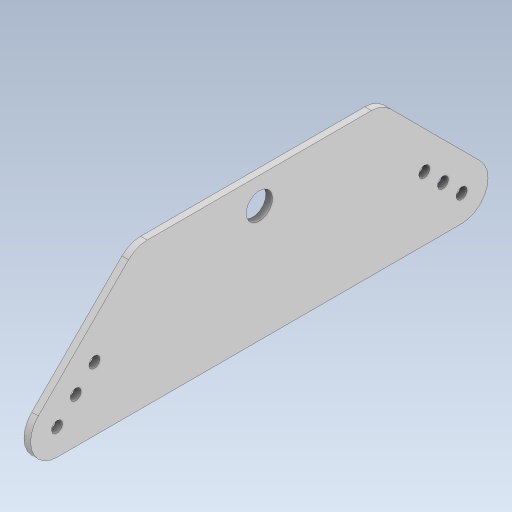
# Autodesk Inventor part: HipPivotPlate
Saved by Autodesk Inventor 2023 (Build 270158000, 158)
## iProperties
Created: 2023-04-06
Part Number: HipPivotPlate
Material: Generic
Document SubType Name: Modeling
Designer: Dave
Density: 1 g/cm^3
Appearance: Default
Author: Dave
Autodesk Inventor part; units mm, degrees
ref_plane "YZ Plane" through (0, 0, 0) normal (1, 0, 0) x (0, 1, 0)
ref_plane "XZ Plane" through (0, 0, 0) normal (0, 1, 0) x (-1, 0, 0)
ref_plane "XY Plane" through (0, 0, 0) normal (0, 0, 1) x (1, 0, 0)
sketch "Sketch1" plane through (0, 0, 0) normal (1, 0, 0) x (0, 1, 0)
  circle A0 centre (0, 0) radius 6.35
  circle A1 centre (-43.3605, -97.242) radius 2.65
  circle A2 centre (-25.4, -79.2815) radius 2.65
  circle A3 centre (-34.3803, 88.2618) radius 2.65
  circle A4 centre (-43.3605, 97.242) radius 2.65
  circle A5 centre (-25.4, 79.2815) radius 2.65
  circle A6 centre (-34.3803, -88.2618) radius 2.65
  line L0 (-34.3803, 88.2618) -> (16.1666, 37.7149) construction
  line L1 (-25.4, -79.2815) -> (-11.4366, -65.3181) construction
  line L2 (-28.0876, 28.0876) -> (0, 0) construction
  line L3 (0, 0) -> (-28.0876, -28.0876) construction
  line L4 (0, 0) -> (18.6115, 0) construction
  line L5 (-34.3803, 106.2223) -> (8.9803, 62.8618)
  line L6 (12.7, 53.8815) -> (12.7, -53.8815)
  line L7 (8.9803, -62.8618) -> (-34.3803, -106.2223)
  line L8 (-52.3408, -106.2223) -> (-52.3408, -106.2223)
  line L9 (-56.0605, -97.242) -> (-56.0605, 97.242)
  line L10 (-52.3408, 106.2223) -> (-52.3408, 106.2223)
  arc A7 (12.7, 53.8815) -> (8.9803, 62.8618) centre (0, 53.8815) ccw
  arc A8 (8.9803, -62.8618) -> (12.7, -53.8815) centre (0, -53.8815) ccw
  arc A9 (-52.3408, -106.2223) -> (-34.3803, -106.2223) centre (-43.3605, -97.242) ccw
  arc A10 (-56.0605, -97.242) -> (-52.3408, -106.2223) centre (-43.3605, -97.242) ccw
  arc A11 (-52.3408, 106.2223) -> (-56.0605, 97.242) centre (-43.3605, 97.242) ccw
  arc A12 (-34.3803, 106.2223) -> (-52.3408, 106.2223) centre (-43.3605, 97.242) ccw
  point P0 (-52.3408, 106.2223)
  dimension "d0" = 12.7
  dimension "d1" = 5.3
  dimension "d2" = 5.3
  dimension "d3" = 5.3
  dimension "d4" = 5.3
  dimension "d5" = 5.3
  dimension "d6" = 5.3
  dimension "d7" = 135
  dimension "d8" = 38.1
  dimension "d9" = 38.1
  dimension "d10" = 25.4
  dimension "d11" = 12.7
  dimension "d12" = 12.7
  dimension "d13" = 25.4
  dimension "d14" = 12.7
  dimension "d15" = 12.7
  dimension "d16" = 12.7
  dimension "d17" = 12.7
  dimension "d18" = 12.7
  dimension "d19" = 45
  dimension "d20" = 12.7
  dimension "d21" = 12.7
  constraints: 22 end point, 13 centre point, 12 point on circle, 12 tangent, 5 equal radius, 4 parallel, 4 point on line, 2 perpendicular, 1 coincident, 1 horizontal, 1 vertical, 2 other
  measures "d0" diameter of A0
  measures "d1" diameter of A1
  measures "d2" diameter of A2
  measures "d3" diameter of A3
  measures "d4" diameter of A4
  measures "d5" diameter of A5
  measures "d6" diameter of A6
  measures "d7" angle of L4 L3
  measures "d8" distance between parallel lines of L2 L0
  measures "d9" distance between parallel lines of L3 L1
  measures "d10" horizontal distance of A5.centre point (0, 0)
  measures "d11" distance of A5.centre L0.start
  measures "d12" distance of L0.start A4.centre
  measures "d13" horizontal distance of L1.start point (0, 0)
  measures "d14" distance of A6.centre L1.start
  measures "d15" distance of A1.centre A6.centre
  measures "d16" distance from line of L5 A5.centre
  measures "d17" distance from line of L10 A4.centre
  measures "d18" distance from line of L6 point (0, 0)
  measures "d19" angle of L6 L5
  measures "d20" distance from line of L9 A4.centre
  measures "d21" radius of A7
extrude "Extrusion1" add sketch "Sketch1" along normal blind 3.175
equation "\"d9\" = d8"
equation "\"d12\" = d11"
equation "\"d13\" = d10"
equation "\"d14\" = d11"
equation "\"d15\" = d11"
body "Solid1"
